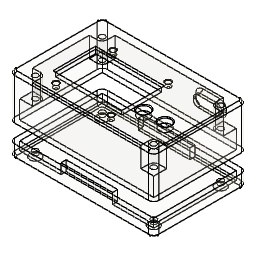
enclosure (Autodesk Fusion 360 design; units mm, degrees)
Autodesk Fusion 360 part; units mm, degrees
sketch "Sketch1" plane through (0, 0, 0) normal (0, 0, 1) x (1, 0, 0) in component "Enclosure-Bottom"
  line L0 (0, 0) -> (50, 0) construction
  line L1 (50, 0) -> (50, 30) construction
  line L2 (50, 30) -> (0, 30) construction
  line L3 (0, 30) -> (0, 0) construction
  line L4 (-1, -1) -> (51, -1)
  line L5 (51, -1) -> (51, 31)
  line L6 (51, 31) -> (-1, 31)
  line L7 (-1, 31) -> (-1, -1)
  line L8 (-1, -3) -> (51, -3)
  line L9 (53, -1) -> (53, 31)
  line L10 (51, 33) -> (-1, 33)
  line L11 (-3, 31) -> (-3, -1)
  arc A0 (53, 31) -> (51, 33) centre (51, 31) ccw
  arc A1 (-1, 33) -> (-3, 31) centre (-1, 31) ccw
  arc A2 (-3, -1) -> (-1, -3) centre (-1, -1) ccw
  arc A3 (51, -3) -> (53, -1) centre (51, -1) ccw
  dimension "d1" = 50
  dimension "d2" = 30
  dimension "d5" = 1
  dimension "d9" = 2
  dimension "d23" = 3
  dimension "d25" = 3
  dimension "d26" = 3
  dimension "d27" = 3
  constraint horizontal L0
  constraint vertical L1
  constraint horizontal L2
  constraint vertical L3
  constraint coincident L0.start L3.end
  constraint parallel L0 L8
  constraint parallel L1 L9
  constraint parallel L2 L10
  constraint parallel L3 L11
  constraint tangent L9 A0
  constraint tangent L10 A0
  constraint tangent L10 A1
  constraint tangent L11 A1
  constraint equal A0 A1
  constraint tangent L11 A2
  constraint tangent L8 A2
  constraint equal A0 A2
  constraint tangent L8 A3
  constraint tangent L9 A3
  constraint equal A0 A3
  measures "d1" distance of L1.end L2.end
  measures "d2" distance of L0.end L1.end
  measures "d9" radius of A0
  measures "d23" distance of L2 L10
  measures "d25" distance of L0 L8
  measures "d26" distance of L3 L11
  measures "d27" distance of L1 L9
extrude "Extrude1" add sketch "Sketch1" against normal blind 2 contours L4 L5 L6 L7 | L8 L9 L10 L11 A0 A1 A2 A3 makes body 1 in component "Enclosure-Bottom"
extrude "Extrude2" add sketch "Sketch1" along normal blind 3.3333 bodies 1 in component "Enclosure-Bottom"
ref_plane "WorkPlane1" through (25, 15, 25.3333) normal (0, 0, 1) x (1, 0, 0)
sketch "Sketch1 (2)" plane through (22.5, 15, 25.3333) normal (0, 0, 1) x (1, 0, 0) in component "Enclosure-Top"
  line L0 (-23.5, -16) -> (28.5, -16)
  line L1 (-23.5, 16) -> (-23.5, -16)
  line L2 (28.5, 16) -> (-23.5, 16)
  line L3 (28.5, -16) -> (28.5, 16)
  line L4 (-23.5, -18) -> (28.5, -18)
  arc A0 (28.5, -18) -> (30.5, -16) centre (28.5, -16) ccw
  line L5 (30.5, -16) -> (30.5, 16)
  line L6 (-25.5, 16) -> (-25.5, -16)
  arc A1 (-25.5, -16) -> (-23.5, -18) centre (-23.5, -16) ccw
  line L7 (28.5, 18) -> (-23.5, 18)
  arc A2 (-23.5, 18) -> (-25.5, 16) centre (-23.5, 16) ccw
  arc A3 (30.5, 16) -> (28.5, 18) centre (28.5, 16) ccw
extrude "Extrude1'" add sketch "Sketch1 (2)" against normal blind 15 separate body makes body 2 in component "Enclosure-Top"
extrude "Extrude2'" add sketch "Sketch1 (2)" along normal blind 2 contours L0 L1 L2 L3 | L4 A0 L5 L6 A1 L7 A2 A3 bodies 2 in component "Enclosure-Top"
fillet "Fillet1" radius 1 8 edges at (53, 15, 27.3333) (52.4142, 32.4142, 27.3333) (25, 33, 27.3333) (-2.4142, 32.4142, 27.3333) (-3, 15, 27.3333) (-2.4142, -2.4142, 27.3333) (25, -3, 27.3333) (52.4142, -2.4142, 27.3333) on bodies 2 in component "Enclosure-Top"
fillet "Fillet1'" radius 1 8 edges at (-3, 15, -2) (-2.4142, 32.4142, -2) (25, 33, -2) (52.4142, 32.4142, -2) (53, 15, -2) (52.4142, -2.4142, -2) (25, -3, -2) (-2.4142, -2.4142, -2) on bodies 1 in component "Enclosure-Bottom"
sketch "Sketch2" plane through (0, 0, 25.3333) normal (0, 0, -1) x (1, 0, 0) in component "Enclosure-Top"
  line L0 (51, 1) -> (-1, 1)
  line L1 (-1, 1) -> (-1, -31)
  line L2 (-1, -31) -> (51, -31)
  line L3 (51, -31) -> (51, 1)
  line L4 (51, -2) -> (-1, -2) construction
  line L5 (2, 1) -> (2, -31) construction
  line L6 (-1, 1) -> (51, 1)
  line L7 (-1, -31) -> (-1, 1)
  line L8 (51, 1) -> (51, -31)
  line L9 (51, -31) -> (-1, -31)
  line L10 (25, 1) -> (25, -31) construction
  line L11 (51, -15) -> (-1, -15) construction
  line L12 (51, -28) -> (-1, -28) construction
  line L13 (48, 1) -> (48, -31) construction
  circle A0 centre (48, -2) radius 1.1
  line L14 (48, -4) -> (51, -4)
  line L15 (46, -2) -> (46, 1)
  arc A1 (46, -2) -> (48, -4) centre (48, -2) ccw
  circle A2 centre (2, -2) radius 1.1
  line L16 (4, -2) -> (4, 1)
  arc A3 (2, -4) -> (4, -2) centre (2, -2) ccw
  line L17 (2, -4) -> (-1, -4)
  circle A4 centre (2, -28) radius 1.1
  line L18 (4, -28) -> (4, -31)
  arc A5 (4, -28) -> (2, -26) centre (2, -28) ccw
  line L19 (2, -26) -> (-1, -26)
  line L20 (48, -26) -> (51, -26)
  circle A6 centre (48, -28) radius 1.1
  arc A7 (48, -26) -> (46, -28) centre (48, -28) ccw
  line L21 (46, -28) -> (46, -31)
  dimension "d28" = 3
  dimension "d29" = 3
  dimension "d30" = 2.2
  dimension "d31" = 4
  constraint coincident L3 L4.start
  constraint coincident L1 L4.end
  constraint perpendicular L1 L4
  constraint coincident L0 L5.start
  constraint coincident L2 L5.end
  constraint perpendicular L2 L5
  constraint midpoint L6 L10.start
  constraint midpoint L9 L10.end
  constraint midpoint L8 L11.start
  constraint midpoint L7 L11.end
  constraint symmetric L4.start L11 L12.start
  constraint symmetric L4.end L11 L12.end
  constraint symmetric L5.start L10 L13.start
  constraint symmetric L5.end L10 L13.end
  constraint coincident L13 A0.centre
  constraint coincident L4 A0.centre
  constraint concentric A0 A1
  constraint coincident L13 L14.start
  constraint coincident L8 L14.end
  constraint tangent L14 A1
  constraint coincident L4 L15.start
  constraint coincident L6 L15.end
  constraint tangent L15 A1
  constraint symmetric L10 A0 A2
  constraint symmetric L10 L14.start A3.start
  constraint symmetric L10 L14.end L17.end
  constraint symmetric L10 L15.start L16.start
  constraint symmetric L10 L15.end L16.end
  constraint symmetric L10 A1 A3
  constraint symmetric L11 A0 A6
  constraint symmetric L11 L14.start L20.start
  constraint symmetric L11 L14.end L20.end
  constraint symmetric L11 L15.start A7.end
  constraint symmetric L11 L15.end L21.end
  constraint symmetric L11 A1 A7
  constraint symmetric L11 A2 A4
  constraint symmetric L11 L16.start L18.start
  constraint symmetric L11 L16.end L18.end
  constraint symmetric L11 A3.start A5.end
  constraint symmetric L11 A3 A5
  constraint symmetric L11 L17.end L19.end
  measures "d28" distance of L0 L4
  measures "d29" distance of L5 L7
  measures "d30" diameter of A0
  measures "d31" diameter of A1
extrude "Extrude3" add sketch "Sketch2" along normal blind 7.8431 contours L0 L3 L6 L8 L14 L15 A1 | L0 L1 L6 L7 L16 A3 L17 | L2 L3 L8 L9 L20 A7 L21 | L1 L2 L7 L9 L18 A5 L19 bodies 2 in component "Enclosure-Top"
sketch "Sketch2 (2)" plane through (0, 0, 0) normal (0, 0, 1) x (-1, 0, 0) in component "Enclosure-Bottom"
  line L0 (1, 1) -> (-51, 1)
  line L1 (-51, 1) -> (-51, -31)
  line L2 (-51, -31) -> (1, -31)
  line L3 (1, -31) -> (1, 1)
  line L4 (1, -31) -> (-51, -31)
  line L5 (-51, -31) -> (-51, 1)
  line L6 (1, 1) -> (1, -31)
  line L7 (-51, 1) -> (1, 1)
  line L8 (-15, -31) -> (-35, -31)
  line L9 (-35, -31) -> (-35, -29)
  line L10 (-35, -29) -> (-15, -29)
  line L11 (-15, -29) -> (-15, -31)
  line L12 (-25, -31) -> (-25, 1) construction
  line L13 (-51, -15) -> (1, -15) construction
  line L14 (-35, -1) -> (-15, -1)
  line L15 (-15, -1) -> (-15, 1)
  line L16 (-35, 1) -> (-35, -1)
  dimension "d34" = 2
  dimension "d35" = 20
  dimension "d36" = 10
  constraint horizontal L8
  constraint vertical L9
  constraint horizontal L10
  constraint vertical L11
  constraint midpoint L4 L12.start
  constraint midpoint L7 L12.end
  constraint midpoint L5 L13.start
  constraint midpoint L6 L13.end
  constraint coincident L4 L8.end
  constraint symmetric L8.start L13 L15.end
  constraint symmetric L8.end L13 L16.start
  constraint symmetric L9.end L13 L14.start
  constraint symmetric L10.end L13 L14.end
  measures "d34" distance of L8.end L9.end
  measures "d35" distance of L9.end L10.end
  measures "d36" distance of L10.end L12
extrude "Extrude3'" add sketch "Sketch2 (2)" along normal blind 4 contours L0 L7 L14 L15 L16 | L2 L4 L8 L9 L10 L11 bodies 1 in component "Enclosure-Bottom"
sketch "Sketch4" plane through (0, 0, -2) normal (0, 0, -1) x (1, 0, 0) in component "Enclosure-Bottom"
  line L0 (-2, 1) -> (-2, -31)
  arc A0 (-2, -31) -> (-1, -32) centre (-1, -31) ccw
  line L1 (-1, -32) -> (51, -32)
  arc A1 (51, -32) -> (52, -31) centre (51, -31) ccw
  line L2 (52, -31) -> (52, 1)
  arc A2 (52, 1) -> (51, 2) centre (51, 1) ccw
  line L3 (51, 2) -> (-1, 2)
  arc A3 (-1, 2) -> (-2, 1) centre (-1, 1) ccw
  circle A4 centre (48, -2) radius 1.1
  circle A5 centre (2, -2) radius 1.1
  circle A6 centre (2, -28) radius 1.1
  circle A7 centre (48, -28) radius 1.1
extrude "Extrude4" cut sketch "Sketch4" against normal up to surface (2 mm away) contours A4 | A5 | A6 | A7 bodies 1 in component "Enclosure-Bottom"
chamfer "Chamfer1" distance 1 angle 45 4 edges at (0.9744, 27.6022, -2) (46.9744, 27.6022, -2) (46.9744, 1.6022, -2) (0.9744, 1.6022, -2) on bodies 1 in component "Enclosure-Bottom"
sketch "Sketch3" plane through (0, 0, 27.3333) normal (0, 0, 1) x (-1, 0, 0) in component "Enclosure-Top"
  line L0 (-52, 1) -> (-52, -31)
  arc A0 (-52, -31) -> (-51, -32) centre (-51, -31) ccw
  line L1 (-51, -32) -> (1, -32)
  arc A1 (1, -32) -> (2, -31) centre (1, -31) ccw
  line L2 (2, -31) -> (2, 1)
  arc A2 (2, 1) -> (1, 2) centre (1, 1) ccw
  line L3 (1, 2) -> (-51, 2)
  arc A3 (-51, 2) -> (-52, 1) centre (-51, 1) ccw
  circle A4 centre (-36.5, -9.6) radius 2.25
  circle A5 centre (-44.8, -9.6) radius 2.25
  line L4 (-6.3775, -5.5187) -> (-32.0775, -5.5187)
  line L5 (-32.0775, -5.5187) -> (-32.0775, -21.0187)
  line L6 (-32.0775, -21.0187) -> (-6.3775, -21.0187)
  line L7 (-6.3775, -21.0187) -> (-6.3775, -5.5187)
extrude "Extrude4'" cut sketch "Sketch3" against normal up to surface (2 mm away) contours A4 | A5 | L4 L5 L6 L7 bodies 2 in component "Enclosure-Top"
chamfer "Chamfer2" distance 0.5 angle 45 4 edges at (6.3775, 13.2687, 27.3333) (19.2275, 21.0187, 27.3333) (32.0775, 13.2687, 27.3333) (19.2275, 5.5187, 27.3333) on bodies 2 in component "Enclosure-Top"
chamfer "Chamfer2" distance 0.3 angle 45 1 edges at (46.8977, 8.7864, 27.3333) on bodies 2 in component "Enclosure-Top"
chamfer "Chamfer2" distance 0.3 angle 45 1 edges at (38.5977, 8.7864, 27.3333) on bodies 2 in component "Enclosure-Top"
sketch "Sketch4 (2)" plane through (0, 0, 25.3333) normal (0, 0, 1) x (-1, 0, 0) in component "Enclosure-Top"
  line L0 (-6.3775, -21.0187) -> (-32.0775, -21.0187)
  line L1 (-32.0775, -21.0187) -> (-32.0775, -5.5187)
  line L2 (-32.0775, -5.5187) -> (-6.3775, -5.5187)
  line L3 (-6.3775, -5.5187) -> (-6.3775, -21.0187)
  circle A0 centre (-36.5, -9.6) radius 2.25
  circle A1 centre (-44.8, -9.6) radius 2.25
  line L4 (-52, 1) -> (-52, -31)
  arc A2 (-52, -31) -> (-51, -32) centre (-51, -31) ccw
  line L5 (-51, -32) -> (1, -32)
  arc A3 (1, -32) -> (2, -31) centre (1, -31) ccw
  line L6 (2, -31) -> (2, 1)
  arc A4 (2, 1) -> (1, 2) centre (1, 1) ccw
  line L7 (1, 2) -> (-51, 2)
  arc A5 (-51, 2) -> (-52, 1) centre (-51, 1) ccw
  circle A6 centre (-8.5275, -25.7187) radius 1
  circle A7 centre (-29.9275, -25.7187) radius 1
  circle A8 centre (-8.5275, -3.5187) radius 1
  circle A9 centre (-29.9275, -3.5187) radius 1
  circle A10 centre (-8.5275, -25.7187) radius 1
  circle A11 centre (-29.9275, -25.7187) radius 1
  circle A12 centre (-8.5275, -3.5187) radius 1
  circle A13 centre (-29.9275, -3.5187) radius 1
  line L8 (-32.0775, -21.0187) -> (-6.3775, -21.0187)
  line L9 (-6.3775, -21.0187) -> (-6.3775, -5.5187)
  line L10 (-6.3775, -5.5187) -> (-32.0775, -5.5187)
  line L11 (-32.0775, -5.5187) -> (-32.0775, -21.0187)
  circle A14 centre (-36.5, -9.6) radius 2.25
  circle A15 centre (-44.8, -9.6) radius 2.25
  line L12 (-2, -4) -> (1, -4)
  line L13 (1, -4) -> (1, -26)
  line L14 (1, -26) -> (-2, -26)
  arc A16 (-2, -26) -> (-4, -28) centre (-2, -28) ccw
  line L15 (-4, -28) -> (-4, -31)
  line L16 (-4, -31) -> (-46, -31)
  line L17 (-46, -31) -> (-46, -28)
  arc A17 (-46, -28) -> (-48, -26) centre (-48, -28) ccw
  line L18 (-48, -26) -> (-51, -26)
  line L19 (-51, -26) -> (-51, -4)
  line L20 (-51, -4) -> (-48, -4)
  arc A18 (-48, -4) -> (-46, -2) centre (-48, -2) ccw
  line L21 (-46, -2) -> (-46, 1)
  line L22 (-46, 1) -> (-4, 1)
  line L23 (-4, 1) -> (-4, -2)
  arc A19 (-4, -2) -> (-2, -4) centre (-2, -2) ccw
  dimension "d49" = 2
  dimension "d50" = 2
  dimension "d51" = 2
  dimension "d52" = 2
  constraint concentric A6 A10
  constraint concentric A7 A11
  constraint concentric A8 A12
  constraint concentric A9 A13
  measures "d49" diameter of A10
  measures "d50" diameter of A11
  measures "d51" diameter of A12
  measures "d52" diameter of A13
extrude "Extrude5" add sketch "Sketch4 (2)" against normal blind 2 contours A6 A10 | A7 A11 | A8 A12 | A9 A13 bodies 2 in component "Enclosure-Top"
fillet "Fillet2" radius 0.2 4 edges at (30.8598, 3.8803, 25.3333) (30.8598, 26.0803, 25.3333) (9.4598, 3.8803, 25.3333) (9.4598, 26.0803, 25.3333) on bodies 2 in component "Enclosure-Top"
chamfer "Chamfer1'" distance 0.5 angle 45 4 edges at (9.4598, 3.1571, 23.3333) (30.8598, 3.1571, 23.3333) (9.4598, 25.3571, 23.3333) (30.8598, 25.3571, 23.3333) on bodies 2 in component "Enclosure-Top"
sketch "Sketch5" plane through (0, 33, 0) normal (0, 1, 0) x (-1, 0, 0) in component "Enclosure-Top"
  line L0 (1, 26.3333) -> (-51, 26.3333)
  line L1 (-51, 26.3333) -> (-51, 10.3333)
  line L2 (-51, 10.3333) -> (1, 10.3333)
  line L3 (1, 10.3333) -> (1, 26.3333)
  line L4 (-39.75, 17.1902) -> (-36.11, 17.1902)
  arc A0 (-36.11, 17.1902) -> (-34.33, 18.9702) centre (-36.11, 18.9702) ccw
  line L5 (-34.33, 18.9702) -> (-34.33, 19.5702)
  arc A1 (-34.33, 19.5702) -> (-36.11, 21.3502) centre (-36.11, 19.5702) ccw
  line L6 (-36.11, 21.3502) -> (-42.49, 21.3502)
  arc A2 (-42.49, 21.3502) -> (-44.27, 19.5702) centre (-42.49, 19.5702) ccw
  line L7 (-44.27, 19.5702) -> (-44.27, 18.9702)
  arc A3 (-44.27, 18.9702) -> (-42.49, 17.1902) centre (-42.49, 18.9702) ccw
  line L8 (-42.49, 17.1902) -> (-39.8, 17.1902)
  line L9 (-39.8, 17.1902) -> (-39.75, 17.1902)
  constraint parallel L4 L9
  constraint tangent L4 A0
  constraint tangent L7 A3
  constraint tangent L5 A1
  constraint tangent A0 L5
  constraint tangent A1 L6
  constraint tangent A2 L7
  constraint tangent L6 A2
  constraint tangent A3 L8
extrude "Extrude6" cut sketch "Sketch5" against normal up to surface (2 mm away) contours L4 A0 L5 A1 L6 A2 L7 A3 L8 L9 bodies 2 in component "Enclosure-Top"
chamfer "Chamfer3" distance 1 angle 45 8 edges at (34.8513, 33, 20.8288) (34.33, 33, 19.2702) (34.8513, 33, 17.7115) (39.3, 33, 17.1902) (43.7487, 33, 17.7115) (44.27, 33, 19.2702) (43.7487, 33, 20.8288) (39.3, 33, 21.3502) on bodies 2 in component "Enclosure-Top"
component "Enclosure-Bottom" placed x (1, 0, 0) y (0, 1, 0) z (0, 0, 1) at (0, 0, 0)
component "Enclosure-Top" placed x (1, 0, 0) y (0, 1, 0) z (0, 0, 1) at (0, 0, 0)
equation "d1 = length"
equation "d2 = width"
equation "wall_thickness = 2 mm"
equation "margin = 1 mm"
equation "d5 = margin"
equation "fillet_radius = 2 mm"
equation "height = 20 mm"
equation "d9 = fillet_radius"
equation "d10 = -wall_thickness"
equation "d12 = height / 6"
equation "d14 = height + wall_thickness"
equation "d15 = -height * ( 3 / 4 )"
equation "d17 = wall_thickness"
equation "d20 = 0.5 * fillet_radius"
equation "d22 = 0.5 * fillet_radius"
equation "d23 = wall_thickness + margin"
equation "d25 = wall_thickness + margin"
equation "d26 = wall_thickness + margin"
equation "d27 = wall_thickness + margin"
equation "d28 = 2 mm + margin"
equation "d29 = 2 mm + margin"
equation "d32 = height / 2.55"
equation "d34 = wall_thickness"
equation "d35 = 10 * wall_thickness"
equation "d36 = ( 10 * wall_thickness ) / 2"
equation "d37 = height / 5"
equation "length = 50 mm"
equation "width = 30 mm"
equation "d53 = -height / 10"
